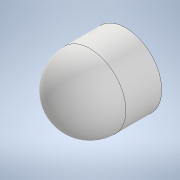
# Autodesk Inventor part: handle_base_rod
Saved by Autodesk Inventor 2021 (Build 250183000, 183)
## iProperties
Created: 2021-07-04
Part Number: handle_base_rod
Material: Generic
Document SubType Name: Modeling
Designer: teh18
Density: 1 g/cm^3
Appearance: Default
Author: teh18
Autodesk Inventor part; units mm, degrees
ref_plane "YZ Plane" through (0, 0, 0) normal (1, 0, 0) x (0, 1, 0)
ref_plane "XZ Plane" through (0, 0, 0) normal (0, 1, 0) x (-1, 0, 0)
ref_plane "XY Plane" through (0, 0, 0) normal (0, 0, 1) x (1, 0, 0)
sketch "Sketch1" plane through (0, 0, 0) normal (0, 0, 1) x (1, 0, 0)
  circle A0 centre (0, 0) radius 6 projected
  circle A1 centre (0, 0) radius 5
  point P0 (0, 0)
  dimension "d0" = 1
  constraints: 1 centre point
  measures "d0" radial gap between concentric circles of A0 A1
extrude "Extrusion1" add sketch "Sketch1" along normal blind 10 and the other way blind 10 contours A1
fillet "Fillet1" radius 5 1 edges at (-5, 0, 10)
body "Solid1"
